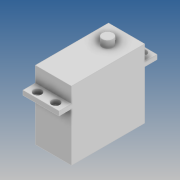
# Autodesk Inventor part: JX PDI-HV5932MG-180 digital servo
Saved by Autodesk Inventor 2020.2 (Build 242310000, 310)
## iProperties
Created: 2020-03-23
Part Number: JX PDI-HV5932MG-180 digital servo
Material: Generic
Document SubType Name: Modeling
Designer: David
Mass: 75 g
Surface Area: 69.2404 cm^2
Volume: 31.4191 cm^3
Density: 2.38709 g/cm^3
Appearance: Smooth - Aqua
Author: David
Autodesk Inventor part; units mm, degrees
ref_plane "YZ Plane" through (0, 0, 0) normal (1, 0, 0) x (0, 1, 0)
ref_plane "XZ Plane" through (0, 0, 0) normal (0, 1, 0) x (-1, 0, 0)
ref_plane "XY Plane" through (0, 0, 0) normal (0, 0, 1) x (1, 0, 0)
sketch "Sketch1" plane through (0, 0, 0) normal (1, 0, 0) x (0, 1, 0)
  line L0 (38, 40.5) -> (0, 40.5)
  line L1 (0, 40.5) -> (0, 0)
  line L2 (0, 0) -> (38, 0)
  line L3 (38, 0) -> (38, 40.5)
  dimension "d0" = 40.5
  dimension "d1" = 38
  constraints: 8 end point, 2 parallel, 1 horizontal, 1 perpendicular
  measures "d0" distance of L0.end L1.end
  measures "d1" distance of L1.end L2.end
extrude "BODY" add sketch "Sketch1" against normal blind 20
sketch "Sketch2" plane through (0, 0, 40.5) normal (0, 0, 1) x (1, 0, 0)
  line L0 (-20, 0) -> (-20, 38) construction
  line L1 (0, 0) -> (-20, 0) construction
  line L2 (0, 27) -> (-20, 27)
  line L3 (-20, 27) -> (-20, 29.5)
  line L4 (-20, 29.5) -> (0, 29.5)
  line L5 (0, 29.5) -> (0, 27)
  dimension "d4" = 27
  dimension "d5" = 2.5
  dimension "d6" = 20
  dimension "d7" = 0
  constraints: 8 end point, 2 parallel, 1 horizontal, 1 perpendicular
  measures "d4" distance between parallel lines of L1 L2
  measures "d5" distance of L4.end L2.start
  measures "d6" distance of L3.end L4.end
  measures "d7" distance between parallel lines of L0 L3
extrude "BRACKET1" add sketch "Sketch2" along normal blind 6.85
sketch "Sketch3" plane through (0, 0, 0) normal (0, 0, -1) x (-1, 0, 0)
  line L0 (0, 0) -> (0, 38) construction
  line L1 (0, 0) -> (20, 0) construction
  line L2 (20, 27) -> (0, 27)
  line L3 (0, 27) -> (0, 29.5)
  line L4 (0, 29.5) -> (20, 29.5)
  line L5 (20, 29.5) -> (20, 27)
  dimension "d10" = 27
  dimension "d11" = 2.5
  dimension "d12" = 0
  dimension "d13" = 20
  constraints: 8 end point, 2 parallel, 1 horizontal, 1 perpendicular
  measures "d10" distance between parallel lines of L1 L2
  measures "d11" distance of L4.end L2.start
  measures "d12" distance between parallel lines of L0 L3
  measures "d13" distance of L3.end L4.end
extrude "BRACKET2" add sketch "Sketch3" along normal blind 6.85
sketch "Sketch4" plane through (-20, 29.5, 40.5) normal (0, 1, 0) x (1, 0, 0)
  line L0 (0, 0) -> (20, 0) construction
  line L1 (20, 0) -> (20, -6.85) construction
  circle A0 centre (5, -3.75) radius 2.25
  circle A1 centre (15, -3.75) radius 2.25
  circle A2 centre (5, 44.25) radius 2.25
  circle A3 centre (15, 44.25) radius 2.25
  line L2 (20, 40.5) -> (20, 47.35) construction
  line L3 (0, 40.5) -> (0, 47.35) construction
  dimension "d16" = 4.5
  dimension "d17" = 4.5
  dimension "d18" = 4.5
  dimension "d19" = 4.5
  dimension "d20" = 48
  dimension "d21" = 48
  dimension "d22" = 10
  dimension "d23" = 5
  dimension "d24" = 5
  dimension "d26" = 10
  dimension "d27" = 3.75
  dimension "d28" = 5
  constraints: 4 centre point
  measures "d16" diameter of A2
  measures "d17" diameter of A3
  measures "d18" diameter of A1
  measures "d19" diameter of A0
  measures "d20" distance of A1.centre A3.centre
  measures "d21" distance of A0.centre A2.centre
  measures "d22" distance of A2.centre A3.centre
  measures "d23" distance from line of L2 A3.centre
  measures "d24" distance from line of L3 A2.centre
  measures "d26" distance of A1.centre A0.centre
  measures "d27" distance from line of L0 A0.centre
  measures "d28" distance from line of L1 A1.centre
extrude "SCREW_HOLES" cut sketch "Sketch4" against normal blind 10
sketch "Sketch5" plane through (0, 38, 40.5) normal (0, 1, 0) x (1, 0, 0)
  line L0 (-20, 0) -> (-20, 40.5) construction
  line L1 (0, 0) -> (-20, 0) construction
  circle A0 centre (-10, 30) radius 3
  dimension "d31" = 6
  dimension "d32" = 30
  dimension "d33" = 10
  constraints: 1 centre point
  measures "d31" diameter of A0
  measures "d32" distance from line of L1 A0.centre
  measures "d33" distance from line of L0 A0.centre
extrude "TORQUE_CENTER" add sketch "Sketch5" along normal blind 4
equation "\"d10\" = d4"
equation "\"d11\" = d5"
equation "\"d13\" = d6"
equation "\"d14\" = d8"
equation "\"d17\" = d16"
equation "\"d18\" = d16"
equation "\"d19\" = d16"
equation "\"d8\" = 6.85"
body "Solid1"
